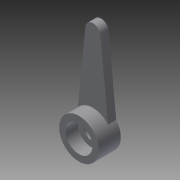
# Autodesk Inventor part: SG90 SingleArm
Saved by Autodesk Inventor 2015 (Build 190159000, 159)
## iProperties
Created: 2020-08-09
Part Number: SG90 SingleArm
Material: 일반
Document SubType Name: Modeling
Designer: penta
Density: 1 g/cm^3
Appearance: 기본값
Author: penta
Autodesk Inventor part; units mm, degrees
ref_plane "YZ Plane" through (0, 0, 0) normal (1, 0, 0) x (0, 1, 0)
ref_plane "XZ Plane" through (0, 0, 0) normal (0, 1, 0) x (-1, 0, 0)
ref_plane "XY Plane" through (0, 0, 0) normal (0, 0, 1) x (1, 0, 0)
sketch "스케치1" plane through (0, 0, 0) normal (0, 1, 0) x (-1, 0, 0)
  circle A0 centre (0, 0) radius 3.4
  dimension "d0" = 6.8
  constraints: 1 centre point, 1 coincident
  measures "d0" diameter of A0
extrude "돌출1" add sketch "스케치1" along normal blind 3.8
hole "구멍1" at (0, 3.8, 0) direction (0, -1, 0) diameter 2.5 end through all
hole "구멍2" at (0, 3.8, 0) direction (0, -1, 0) diameter 4.6 depth 1.1
hole "구멍3" at (0, 0, 0) direction (0, 1, 0) diameter 4.6 depth 2.1
sketch "스케치2" plane through (0, 3.8, 0) normal (0, 1, 0) x (1, 0, 0)
  line L0 (0, 3.4) -> (0, -16)
  line L1 (-2.6, -2.1909) -> (-1.2931, -14.8337)
  arc A0 (0, 3.4) -> (-2.6, -2.1909) centre (0, 0) ccw
  arc A1 (-1.2931, -14.8337) -> (0, -16) centre (0, -14.7) ccw
  line L2 (2.6, -2.1909) -> (1.2931, -14.8337)
  arc A2 (2.6, -2.1909) -> (0, 3.4) centre (0, 0) ccw
  arc A3 (0, -16) -> (1.2931, -14.8337) centre (0, -14.7) ccw
  arc A4 (-2.6, -2.1909) -> (2.6, -2.1909) centre (0, 0) ccw
  dimension "d34" = 19.4
  constraints: 10 point on circle, 6 end point, 5 centre point, 2 coincident, 2 symmetric about line, 1 point on line, 1 tangent, 1 vertical, 2 other
  measures "d34" distance of L0.start L0.end
extrude "돌출2" add sketch "스케치2" against normal blind 1.4 contours A4 L2 A3 L0 | L0 A1 L1 A4
